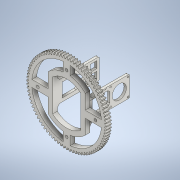
# Autodesk Inventor part: Spur Gear2
Saved by Autodesk Inventor 2020 (Build 240168000, 168)
## iProperties
CustomPartVersion: 1
Created: 2019-04-12
Part Number: Spur Gear2
Material: Steel
Document SubType Name: Modeling
Designer: Connor
Categories: <?xml version="1.0" encoding="UTF-16"?> <MemberInstance><Categories><FamilyTemplate><FamilyTemplateParameter ValueType="xs:double" Id="1" ObjectReferenceKey="da_z" ObjectType="kUserParameterObject"/><FamilyTemplateParameter ValueType="xs:double" Id="2" ObjectReferenceKey="da_b" ObjectType="kUserParameterObject"/><FamilyTemplateParameter ValueType="xs:double" Id="3" ObjectReferenceKey="da_beta" ObjectType="kUserParameterObject"/><FamilyTemplateParameter ValueType="xs:double" Id="4" ObjectReferenceKey="da_da" ObjectType="kUserParameterObject"/><FamilyTemplateParameter ValueType="xs:double" Id="5" ObjectReferenceKey="da_aw" ObjectType="kUserParameterObject"/><FamilyTemplateParameter ValueType="xs:string" Id="6" ObjectReferenceKey="EAIAABAAAAC/AAAAAAAAAIAAAAAAAAAA" ObjectType="83910656" SubObjectId="SurfaceGeometry"/></FamilyTemplate><ParamToTemplateMap><ParamToTemplate CategoryParameter="//CategoryParameter[@InternalName='046C89C9-8512-4d59-83FE-43B91F4F132A']" TemplateParameter="1"/><ParamToTemplate CategoryParameter="//CategoryParameter[@InternalName='2552DF32-E462-4b46-AEBF-C6C7768E72AC']" TemplateParameter="2"/><ParamToTemplate CategoryParameter="//CategoryParameter[@InternalName='C9EE641D-15FC-4fae-A226-E94C4372FDD7']" TemplateParameter="3"/><ParamToTemplate><ParamToTemplate CategoryParameter="//CategoryParameter[@InternalName='00B6519A-459B-49c7-AD84-2E56D39A5744']" ConstantValue="0.000000"/></ParamToTemplate><ParamToTemplate><ParamToTemplate CategoryParameter="//CategoryParameter[@InternalName='04B31F0E-C7A6-4894-AA32-9629BEFACF47']" ConstantValue="1.000000"/></ParamToTemplate><ParamToTemplate><ParamToTemplate CategoryParameter="//CategoryParameter[@InternalName='43CBEC2E-7847-49e7-A936-2F7889FCB2D9']" ConstantValue="0.250000"/></ParamToTemplate><ParamToTemplate><ParamToTemplate CategoryParameter="//CategoryParameter[@InternalName='B1EFC894-105D-4ebd-86BF-FA20ED196853']" ConstantValue="0.350000"/></ParamToTemplate><ParamToTemplate><ParamToTemplate CategoryParameter="//CategoryParameter[@InternalName='51175063-3D10-4879-93E8-6246FE8B403D']" ConstantValue="2061532430.657340"/></ParamToTemplate><ParamToTemplate><ParamToTemplate CategoryParameter="//CategoryParameter[@InternalName='A3A52E27-4454-46a9-B0BD-C932399B70AF']" ConstantValue="0.300000"/></ParamToTemplate><ParamToTemplate><ParamToTemplate CategoryParameter="//CategoryParameter[@InternalName='91B76062-C214-41d9-B1B9-14D2AB99603D']" ConstantValue="0.254000"/></ParamToTemplate><ParamToTemplate><ParamToTemplate CategoryParameter="//CategoryParameter[@InternalName='374E806E-8B8A-4dda-A9AA-1039D6500AD2']" ConstantValue="3.937008"/></ParamToTemplate><ParamToTemplate><ParamToTemplate CategoryParameter="//CategoryParameter[@InternalName='2D373A89-B862-43d6-8D0B-0CBF12AB9F6C']" ConstantValue="0.349066"/></ParamToTemplate><ParamToTemplate CategoryParameter="//CategoryParameter[@InternalName='37777632-D6A2-4fac-9D53-DB8ACD95C989']" TemplateParameter="4"/><ParamToTemplate CategoryParameter="//CategoryParameter[@InternalName='FD1017F1-B727-4f7e-9707-0F86F1FF9423']" TemplateParameter="5"/><ParamToTemplate><ParamToTemplate CategoryParameter="//CategoryParameter[@InternalName='9E1B4470-B2D3-4ff1-B813-535BB4CDF51A']" ConstantValue="3523220.976809"/></ParamToTemplate><ParamToTemplate><ParamToTemplate CategoryParameter="//CategoryParameter[@InternalName='F8452263-BFF6-458c-9FB1-07C4B99E95CD']" ConstantValue="11397033.805607"/></ParamToTemplate><ParamToTemplate><ParamToTemplate CategoryParameter="//CategoryParameter[@InternalName='3E3BB259-FD49-497f-8171-6EBC954A3479']" ConstantValue="2.000000"/></ParamToTemplate><ParamToTemplate CategoryParameter="//CategoryParameter[@InternalName='27C3BAF2-7550-4e4b-AE2C-0DB134B7D9B7']" TemplateParameter="6"/></ParamToTemplateMap><Category DisplayName="Gear" InternalName="DC85795E-93AB-48d5-8EEE-5A27447B64BD" Mnemonic="Gear"><CategoryParameter DisplayName="z" InternalName="046C89C9-8512-4d59-83FE-43B91F4F132A" Mnemonic="z"/><CategoryParameter DisplayName="b" InternalName="2552DF32-E462-4b46-AEBF-C6C7768E72AC" Mnemonic="b"/><CategoryParameter DisplayName="||b|" InternalName="C9EE641D-15FC-4fae-A226-E94C4372FDD7" Mnemonic="beta"/><CategoryParameter DisplayName="x" InternalName="00B6519A-459B-49c7-AD84-2E56D39A5744" Mnemonic="x"/><CategoryParameter DisplayName="a*" InternalName="04B31F0E-C7A6-4894-AA32-9629BEFACF47" Mnemonic="a"/><CategoryParameter DisplayName="c*" InternalName="43CBEC2E-7847-49e7-A936-2F7889FCB2D9" Mnemonic="c"/><CategoryParameter DisplayName="r|.f|*" InternalName="B1EFC894-105D-4ebd-86BF-FA20ED196853" Mnemonic="rf"/><CategoryParameter DisplayName="E" InternalName="51175063-3D10-4879-93E8-6246FE8B403D" Mnemonic="E"/><CategoryParameter DisplayName="||m|" InternalName="A3A52E27-4454-46a9-B0BD-C932399B70AF" Mnemonic="mi"/><Category DisplayName="SpurGear" InternalName="26C5A22E-A91E-4dfd-A3B3-23CCAFAE1764" Mnemonic="SpurGear"><CategoryParameter DisplayName="m" InternalName="91B76062-C214-41d9-B1B9-14D2AB99603D" Mnemonic="m"/><CategoryParameter DisplayName="P" InternalName="374E806E-8B8A-4dda-A9AA-1039D6500AD2" Mnemonic="PP"/><CategoryParameter DisplayName="||a|" InternalName="2D373A89-B862-43d6-8D0B-0CBF12AB9F6C" Mnemonic="alpha"/><CategoryParameter DisplayName="d|.a|" InternalName="37777632-D6A2-4fac-9D53-DB8ACD95C989" Mnemonic="da"/><CategoryParameter DisplayName="a|.w|" InternalName="FD1017F1-B727-4f7e-9707-0F86F1FF9423" Mnemonic="aw"/><CategoryParameter DisplayName="||s||.Flim|" InternalName="9E1B4470-B2D3-4ff1-B813-535BB4CDF51A" Mnemonic="sFlim"/><CategoryParameter DisplayName="||s||.Hlim|" InternalName="F8452263-BFF6-458c-9FB1-07C4B99E95CD" Mnemonic="sHlim"/><CategoryParameter DisplayName="type" InternalName="3E3BB259-FD49-497f-8171-6EBC954A3479" Mnemonic="type"/><CategoryParameter DisplayName="PitchDiameter" InternalName="27C3BAF2-7550-4e4b-AE2C-0DB134B7D9B7" Mnemonic="IDS_PITCHDIAM"/></Category></Category></Categories></MemberInstance>
Density: 1 g/cm^3
Appearance: Steel
Author: Connor
Autodesk Inventor part; units mm, degrees
sketch "Sketch1" plane through (0, 0, 0) normal (0, 0, 1) x (1, 0, 0)
  circle A0 centre (0, 0) radius 109.22
  dimension "d0" = 218.44
  constraints: 1 centre point
  measures "d0" diameter of A0
extrude "Extrusion1" add sketch "Sketch1" along normal blind 12.7
sketch "Sketch2" plane through (0, 0, 0) normal (0, 0, -1) x (-1, 0, 0)
  circle A0 centre (0, 0) radius 109.22 projected
  circle A1 centre (0, 0) radius 106.68
  dimension "d3" = 213.36
  constraints: 1 centre point, 1 coincident
  measures "d3" diameter of A1
surface extrude "Pitch Diameter" sketch "Sketch2" against normal through all shown no curves A1
ref_plane "Work Plane1" through (0, 0, 0) normal (1, 0, 0) x (0, 1, 0)
ref_plane "Work Plane2" through (0, 0, 0) normal (0.9993007, 0.0373912, 0) x (0, 0, 1)
ref_plane "Work Plane3" through (0, 0, 6.35) normal (0, 0, -1) x (-1, 0, 0)
spur gear teeth "Spur Gear" teeth 84 pitch diameter 213.36 tip diameter 218.44 root diameter 207.01 face width 12.7 start plane through (0, 0, 0) normal (0, 0, -1) x (-1, 0, 0)
sketch "Sketch3" plane through (0, 0, 12.7) normal (0, 0, 1) x (1, 0, 0)
  circle A0 centre (0, 0) radius 58.1025
  circle A1 centre (78.6638, 0) radius 3.81
  circle A2 centre (-78.6638, 0) radius 3.81
  circle A3 centre (0, 0) radius 73.025 construction
  arc A4 (20.1928, 101.5162) -> (18.2911, 101.876) centre (0, 0) ccw projected
  dimension "d66" = 116.205
  dimension "d67" = 146.05
  dimension "d68" = 7.62
  dimension "d69" = 7.62
  dimension "d70" = 1.8288
  dimension "d71" = 1.8288
  constraints: 4 centre point, 2 horizontal alignment, 1 coincident, 1 concentric
  measures "d66" diameter of A0
  measures "d67" diameter of A3
  measures "d68" diameter of A2
  measures "d69" diameter of A1
extrude "Extrusion8" cut sketch "Sketch3" against normal blind 25.4
sketch "Sketch9" plane through (0, 0, 12.7) normal (0, 0, 1) x (1, 0, 0)
  circle A0 centre (0, 0) radius 58.1025 projected
  line L0 (-38.1, 43.8667) -> (-38.1, -43.8667)
  line L1 (38.1, 43.8667) -> (38.1, -43.8667)
  line L2 (-38.1, 28.2) -> (-44.45, 28.2)
  line L3 (-44.45, 28.2) -> (-44.45, -28.2)
  line L4 (-44.45, -28.2) -> (-38.1, -28.2)
  line L5 (-38.1, -28.2) -> (-38.1, 28.2)
  line L6 (-38.1, 28.2) -> (0, 0) construction
  line L7 (0, 0) -> (-38.1, -28.2) construction
  line L8 (38.1, 28.2) -> (44.45, 28.2)
  line L9 (44.45, 28.2) -> (44.45, -28.2)
  line L10 (44.45, -28.2) -> (38.1, -28.2)
  line L11 (38.1, -28.2) -> (38.1, 28.2)
  dimension "d75" = 56.4
  dimension "d76" = 6.35
  dimension "d77" = 76.2
  constraints: 24 end point, 4 equal length, 4 parallel, 4 point on circle, 2 horizontal, 2 perpendicular, 2 point on line, 2 vertical, 1 collinear
  measures "d75" distance of L2.end L3.end
  measures "d76" distance of L2.start L2.end
  measures "d77" distance between parallel lines of L1 L0
extrude "Extrusion9" add sketch "Sketch9" against normal up to surface (12.7 mm away) contours A0 L1 L10 L9 L8 | L0 L2 L3 L4 A0 | L8 L9 L10 L1 | L0 L4 L3 L2
extrude "Extrusion10" add sketch "Sketch9" against normal blind 127 contours L8 L9 L10 L1 | L0 L4 L3 L2
sketch "Sketch10" plane through (44.45, -28.2, 0) normal (1, 0, 0) x (0, 0, -1)
  line L0 (0, 0) -> (114.3, 0) construction
  line L1 (57.9, 0) -> (57.9, 56.4) construction
  line L2 (0, 56.4) -> (114.3, 56.4) construction
  line L3 (114.3, 56.4) -> (114.3, 0) construction
  line L4 (57.9, 0) -> (114.3, 56.4) construction
  line L5 (57.9, 56.4) -> (114.3, 0) construction
  circle A0 centre (62.53, 4.63) radius 2.25
  circle A1 centre (62.53, 51.77) radius 2.25
  circle A2 centre (109.67, 4.63) radius 2.25
  circle A3 centre (109.67, 51.77) radius 2.25
  circle A4 centre (86.1, 28.2) radius 19.3
  point P0 (0, 28.2)
  dimension "d82" = 56.4
  dimension "d83" = 4.5
  dimension "d85" = 47.14
  dimension "d86" = 38.6
  constraints: 6 end point, 6 point on line, 5 centre point, 3 equal radius, 2 vertical alignment, 1 horizontal alignment, 1 midpoint, 1 vertical
  measures "d82" distance between parallel lines of L3 L1
  measures "d83" diameter of A0
  measures "d85" distance of A1.centre A0.centre
  measures "d86" diameter of A4
extrude "Extrusion11" cut sketch "Sketch10" against normal up to surface (6.35 mm away)
sketch "Sketch11" plane through (-44.45, -28.2, 0) normal (-1, 0, 0) x (0, 0, 1)
  line L0 (0, 56.4) -> (-114.3, 56.4) construction
  line L1 (-57.9, 56.4) -> (-57.9, 0) construction
  line L2 (0, 0) -> (-114.3, 0) construction
  line L3 (-114.3, 0) -> (-114.3, 56.4) construction
  line L4 (0, 0) -> (-114.3, 0) construction
  line L5 (-57.9, 56.4) -> (-114.3, 0) construction
  line L6 (0, 56.4) -> (-114.3, 56.4) construction
  line L7 (-114.3, 56.4) -> (-57.9, 0) construction
  circle A0 centre (-86.1, 28.2) radius 2.6035
  point P0 (0, 28.2)
  dimension "d89" = 56.4
  dimension "d90" = 5.207
  constraints: 6 end point, 2 point on line, 1 centre point, 1 midpoint, 1 vertical
  measures "d89" distance between parallel lines of L3 L1
  measures "d90" diameter of A0
extrude "Extrusion12" cut sketch "Sketch11" against normal up to surface (6.35 mm away)
fillet "Fillet3" radius 3.175 4 edges at (41.275, 28.2, -114.3) (41.275, -28.2, -114.3) (-41.275, -28.2, -114.3) (-41.275, 28.2, -114.3)
sketch "Sketch12" plane through (0, 0, 12.7) normal (0, 0, 1) x (1, 0, 0)
  arc A0 (-38.1, -43.8667) -> (38.1, -43.8667) centre (0, 0) ccw projected
  line L0 (38.1, 43.8667) -> (38.1, -43.8667) projected
  arc A1 (38.1, 43.8667) -> (-38.1, 43.8667) centre (0, 0) ccw projected
  line L1 (-38.1, -43.8667) -> (-38.1, 43.8667) projected
  arc A2 (-50.8, -49.3189) -> (50.8, -49.3189) centre (0, 0) ccw
  line L2 (-50.8, -49.3189) -> (-50.8, 49.3189)
  arc A3 (50.8, 49.3189) -> (-50.8, 49.3189) centre (0, 0) ccw
  line L3 (50.8, 49.3189) -> (50.8, -49.3189)
  circle A4 centre (0, 0) radius 95.1738
  line L4 (50.8, 34.55) -> (50.8, -34.55) construction
  line L5 (50.8, -9.525) -> (94.696, -9.525)
  line L6 (50.8, 9.525) -> (94.696, 9.525)
  line L7 (-50.8, -34.55) -> (-50.8, 34.55) construction
  line L8 (-50.8, -9.525) -> (-94.696, -9.525)
  line L9 (-50.8, 9.525) -> (-94.696, 9.525)
  circle A5 centre (78.6638, 0) radius 3.81 construction
  line L10 (9.525, -94.696) -> (9.525, -70.1589)
  line L11 (-9.525, -70.1589) -> (-9.525, -94.696)
  line L12 (9.525, 70.1589) -> (9.525, 94.696)
  line L13 (-9.525, 70.1589) -> (-9.525, 94.696)
  dimension "d97" = 12.7
  dimension "d98" = 19.05
  dimension "d99" = 12.7
  dimension "d100" = 19.05
  constraints: 20 end point, 8 point on circle, 6 equal length, 4 point on line, 3 perpendicular, 2 centre point, 2 parallel, 2 vertical, 1 coincident, 1 horizontal, 13 other
  measures "d97" radial gap between concentric circles of A0 A2
  measures "d98" distance between parallel lines of L6 L5
  measures "d100" distance between parallel lines of L11 L10
extrude "Extrusion13" cut sketch "Sketch12" against normal up to surface (12.7 mm away) contours A2 L11 A4 L8 L2 | A2 L3 L5 A4 L10 | L9 A4 L13 A3 L2 | L3 A3 L12 A4 L6
sketch "Sketch15" plane through (38.1, 28.2, 0) normal (0, 1, 0) x (1, 0, 0)
  line L0 (0, 111.125) -> (6.35, 111.125) projected
  line L1 (0, 0) -> (0, 111.125) projected
  line L2 (6.35, 0) -> (0, 0) projected
  line L3 (6.35, 0) -> (6.35, 111.125) projected
  line L4 (-82.55, 111.125) -> (-76.2, 111.125) projected
  line L5 (-82.55, 0) -> (-82.55, 111.125) projected
  line L6 (-76.2, 0) -> (-82.55, 0) projected
  line L7 (-76.2, 0) -> (-76.2, 111.125) projected
  line L8 (6.35, 0) -> (6.35, 111.125) projected
  line L9 (6.35, 0) -> (12.7, 0)
  line L10 (12.7, 0) -> (6.35, 50.8)
  line L11 (-82.55, 0) -> (-88.9, 0)
  line L12 (-132.796, 0) -> (-47.625, 0) projected
  line L13 (-88.9, 0) -> (-82.55, 50.8)
  line L14 (-82.55, 0) -> (-82.55, 111.125) projected
  point P0 (-38.1, 0)
  dimension "d103" = 6.35
  dimension "d104" = 50.8
  dimension "d105" = 6.35
  constraints: 8 end point, 3 point on line, 1 horizontal, 1 horizontal alignment
  measures "d103" distance of L2.start L9.end
  measures "d104" distance from line of L2 L10.end
  measures "d105" distance of L5.start L11.end
extrude "Extrusion14" add sketch "Sketch15" against normal up to surface (56.4 mm away) contours L10 L9 L3 | L5 L11 L13
sketch "Sketch16" plane through (0, 0, -114.3) normal (0, 0, -1) x (-1, 0, 0)
  line L0 (-44.45, 25.025) -> (-38.1, 25.025) projected
  line L1 (-44.45, 25.025) -> (-50.8, 25.025)
  line L2 (-50.8, 25.025) -> (-50.8, -25.025)
  line L3 (-50.8, -25.025) -> (-44.45, -25.025)
  line L4 (-44.45, -25.025) -> (-44.45, 25.025)
  line L5 (-38.1, -25.025) -> (-44.45, -25.025) projected
  line L6 (-50.8, 28.2) -> (-50.8, 9.525) projected
  line L7 (44.45, -28.2) -> (44.45, 28.2) projected
  line L8 (44.45, 25.025) -> (50.8, 25.025)
  line L9 (50.8, 25.025) -> (50.8, -25.025)
  line L10 (50.8, -25.025) -> (44.45, -25.025)
  line L11 (44.45, -25.025) -> (44.45, 25.025)
  line L12 (50.8, -28.2) -> (50.8, -9.525) projected
  point P0 (0, 0)
  constraints: 16 end point, 5 collinear, 4 parallel, 2 horizontal, 2 perpendicular, 1 point on line
extrude "Extrusion15" cut sketch "Sketch16" against normal up to surface (114.3 mm away)
chamfer "Chamfer2" distance 6.35 angle 45 6 edges at (44.45, 0, 0) (-44.45, 0, 0) (-44.45, 28.2, 0) (-44.45, -28.2, 0) (44.45, -28.2, 0) (44.45, 28.2, 0)
sketch "Sketch17" plane through (-44.45, -25.025, -114.3) normal (-1, 0, 0) x (0, 0, 1)
  circle A0 centre (28.2, 25.025) radius 2.6035 projected
  circle A1 centre (28.2, 25.025) radius 8.9535
  line L0 (107.95, 50.05) -> (107.95, 0) projected
  line L1 (63.5, 50.05) -> (107.95, 50.05) projected
  line L2 (63.5, 50.05) -> (63.5, 53.225) projected
  line L3 (63.5, 53.225) -> (3.175, 53.225) projected
  arc A2 (3.175, 53.225) -> (0, 50.05) centre (3.175, 50.05) ccw projected
  line L4 (0, 0) -> (0, 50.05) projected
  arc A3 (0, 0) -> (3.175, -3.175) centre (3.175, 0) ccw projected
  line L5 (63.5, -3.175) -> (3.175, -3.175) projected
  line L6 (63.5, -3.175) -> (63.5, 0) projected
  line L7 (63.5, 0) -> (107.95, 0) projected
  circle A4 centre (28.2, 25.025) radius 2.6035 projected
  line L8 (6.35, 46.875) -> (57.15, 46.875)
  line L9 (57.15, 46.875) -> (57.15, 43.7)
  line L10 (57.15, 43.7) -> (101.6, 43.7)
  line L11 (101.6, 43.7) -> (101.6, 6.35)
  line L12 (101.6, 6.35) -> (57.15, 6.35)
  line L13 (57.15, 6.35) -> (57.15, 3.175)
  line L14 (57.15, 3.175) -> (6.35, 3.175)
  line L15 (6.35, 3.175) -> (6.35, 46.875)
  line L16 (31.375, 16.6533) -> (31.375, 3.175)
  line L17 (25.025, 16.6533) -> (25.025, 3.175)
  line L18 (31.375, 46.875) -> (31.375, 33.3967)
  line L19 (25.025, 46.875) -> (25.025, 33.3967)
  line L20 (19.8283, 28.2) -> (6.35, 28.2)
  line L21 (19.8283, 21.85) -> (6.35, 21.85)
  line L22 (28.2, 25.025) -> (57.15, 43.7) construction
  line L23 (28.2, 25.025) -> (57.15, 6.35) construction
  line L24 (56.2148, 46.875) -> (33.5138, 32.2311)
  line L25 (63.0071, 43.7) -> (36.956, 26.895)
  line L26 (63.0071, 6.35) -> (36.956, 23.155)
  line L27 (33.5138, 17.8189) -> (56.2148, 3.175)
  point P0 (114.3, 25.025)
  dimension "d113" = 6.35
  dimension "d114" = 6.35
  dimension "d115" = 6.35
  dimension "d116" = 6.35
  dimension "d119" = 3.175
  dimension "d120" = 3.175
  constraints: 40 end point, 10 point on line, 6 equal length, 4 parallel, 4 vertical, 2 perpendicular, 19 other
  measures "d114" distance between parallel lines of L3 L8
  measures "d115" distance between parallel lines of L17 L16
  measures "d116" distance between parallel lines of L21 L20
  measures "d119" distance between parallel lines of L22 L25
  measures "d120" distance between parallel lines of L22 L24
extrude "Extrusion17" cut sketch "Sketch17" against normal up to surface (6.35 mm away) contours A1 L25 L10 L11 L12 L26 | A1 L18 L8 L24 | L27 L14 L16 A1 | A1 L20 L15 L8 L19 | L17 L14 L15 L21 A1
sketch "Sketch18" plane through (44.45, -25.025, -114.3) normal (1, 0, 0) x (0, 0, -1)
  circle A0 centre (-51.77, 1.455) radius 2.25 projected
  circle A1 centre (-28.2, 25.025) radius 19.3 projected
  circle A2 centre (-4.63, 1.455) radius 2.25 projected
  line L0 (-107.95, 0) -> (-107.95, 50.05) projected
  line L1 (-63.5, 0) -> (-107.95, 0) projected
  line L2 (-63.5, 0) -> (-63.5, -3.175) projected
  line L3 (-63.5, -3.175) -> (-3.175, -3.175) projected
  arc A3 (-3.175, -3.175) -> (0, 0) centre (-3.175, 0) ccw projected
  line L4 (0, 50.05) -> (0, 0) projected
  arc A4 (0, 50.05) -> (-3.175, 53.225) centre (-3.175, 50.05) ccw projected
  line L5 (-63.5, 53.225) -> (-3.175, 53.225) projected
  line L6 (-63.5, 53.225) -> (-63.5, 50.05) projected
  line L7 (-63.5, 50.05) -> (-107.95, 50.05) projected
  circle A5 centre (-4.63, 48.595) radius 2.25 projected
  circle A6 centre (-51.77, 48.595) radius 2.25 projected
  line L8 (-101.6, 6.35) -> (-101.6, 43.7)
  line L9 (-101.6, 43.7) -> (-57.15, 43.7)
  line L10 (-57.15, 43.7) -> (-57.15, 46.875)
  line L11 (-57.15, 46.875) -> (-6.35, 46.875)
  line L12 (-6.35, 46.875) -> (-6.35, 3.175)
  line L13 (-6.35, 3.175) -> (-57.15, 3.175)
  line L14 (-57.15, 3.175) -> (-57.15, 6.35)
  line L15 (-57.15, 6.35) -> (-101.6, 6.35)
  circle A7 centre (-51.77, 1.455) radius 8.6
  circle A8 centre (-51.77, 48.595) radius 8.6
  circle A9 centre (-4.63, 48.595) radius 8.6
  circle A10 centre (-4.63, 1.455) radius 8.6
  circle A11 centre (-28.2, 25.025) radius 25.65
  line L16 (-53.85, 9.7997) -> (-53.85, 40.2503)
  line L17 (-59.0372, 6.35) -> (-53.85, 11.5372)
  line L18 (-53.85, 38.5128) -> (-59.0372, 43.7)
  line L19 (-63.0071, 43.7) -> (-101.6, 43.7) projected
  point P0 (-114.3, 25.025)
  point P1 (-59.0372, 43.7)
  dimension "d123" = 6.35
  dimension "d124" = 6.35
  dimension "d125" = 6.35
  dimension "d126" = 135
  dimension "d127" = 135
  constraints: 22 end point, 4 point on line, 3 centre point, 1 equal radius, 1 tangent, 1 vertical, 16 other
  measures "d123" distance between parallel lines of L1 L15
  measures "d125" radial gap between concentric circles of A1 A11
  measures "d126" angle of L16 L17
  measures "d127" angle of L16 L18
extrude "Extrusion18" cut sketch "Sketch18" against normal up to surface (6.35 mm away) contours L16 L17 L15 L8 L9 L18
ref_plane "Work Plane5" through (0, 0, -7.62) normal (0, 0, -1) x (-1, 0, 0)
sketch "Sketch20" plane through (0, 0, 12.7) normal (0, 0, 1) x (1, 0, 0)
  circle A0 centre (0, 78.6638) radius 3.81
  circle A1 centre (0, -78.6638) radius 3.81
  circle A2 centre (-78.6638, 0) radius 3.81 projected
  circle A3 centre (78.6638, 0) radius 3.81 projected
  point P0 (0, 0)
  dimension "d131" = 157.3276
  dimension "d132" = 78.6638
  constraints: 2 centre point, 2 equal radius, 2 vertical alignment
  measures "d131" distance of A1.centre A0.centre
  measures "d132" distance of point (0, 0) A1.centre
extrude "Extrusion19" cut sketch "Sketch20" against normal up to surface (12.7 mm away) contours A0 | A1
equation "\"d0\" = da_da"
equation "\"d1\" = da_b"
equation "\"d3\" = da_dw"
equation "\"d15\" = da_aw"
equation "\"d19\" = da_aw"
equation "\"da_da\" = 218.44"
equation "\"da_b\" = 12.7"
equation "\"da_dw\" = 213.36"
equation "\"da_aw\" = 124.46"
body "Solid1"
body "Srf1"
